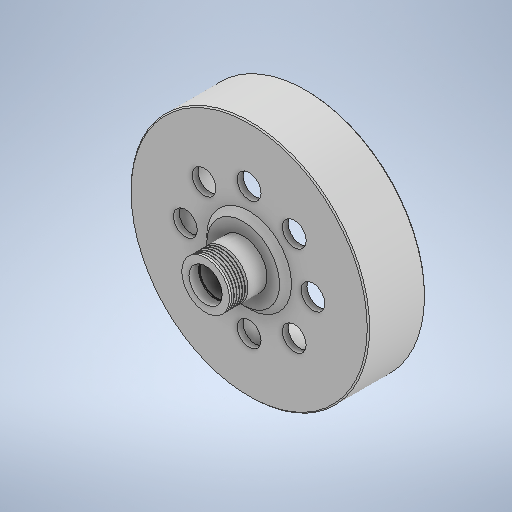
# Autodesk Inventor part: 59-01-002-B
Saved by Autodesk Inventor 2025.2 (Build 292293000, 293)
## iProperties
Created: 2024-11-28
Part Number: 59-01-002-B
Material: Generic
Document SubType Name: Modeling
Designer: Zvonko.Gabric
Density: 1 g/cm^3
Appearance: Default
Author: Zvonko.Gabric
Autodesk Inventor part; units mm, degrees
ref_plane "YZ Plane" through (0, 0, 0) normal (1, 0, 0) x (0, 1, 0)
ref_plane "XZ Plane" through (0, 0, 0) normal (0, 1, 0) x (-1, 0, 0)
ref_plane "XY Plane" through (0, 0, 0) normal (0, 0, 1) x (1, 0, 0)
sketch "Sketch1" plane through (0, 0, 0) normal (0, 1, 0) x (-1, 0, 0)
  line L0 (0, 0) -> (0, 81.9907)
  line L1 (100, 48) -> (100, 0)
  line L2 (35.5, 48) -> (100, 48)
  line L3 (30.5, 53) -> (35.5, 48)
  line L4 (20, 53) -> (30.5, 53)
  line L5 (20, 68.9767) -> (20, 53)
  line L6 (18.0006, 69.7045) -> (20, 68.9767)
  line L7 (19.8684, 70.9857) -> (18.0006, 70.3059)
  line L8 (18.0006, 72.0414) -> (19.8684, 71.3616)
  line L9 (19.8684, 73.3227) -> (18.0006, 72.6428)
  line L10 (18.0006, 74.3784) -> (19.8684, 73.6986)
  line L11 (19.8684, 75.6597) -> (18.0006, 74.9798)
  line L12 (18.0006, 76.7154) -> (19.8684, 76.0355)
  line L13 (19.8684, 77.9966) -> (18.0006, 77.3168)
  line L14 (18.0006, 79.0523) -> (19.8684, 78.3725)
  line L15 (19.8684, 80.3336) -> (18.0006, 79.6537)
  line L16 (18.0006, 81.3893) -> (19.8684, 80.7095)
  line L17 (0, 81.9907) -> (18.0006, 81.9907)
  line L18 (0, 0) -> (0, 81.9907)
  line L19 (100, 0) -> (0, 0)
  arc A0 (18.0006, 70.3059) -> (18.0006, 69.7045) centre (18.11, 70.0052) ccw
  arc A1 (19.8684, 70.9857) -> (19.8684, 71.3616) centre (19.8, 71.1737) ccw
  arc A2 (18.0006, 72.6428) -> (18.0006, 72.0414) centre (18.11, 72.3421) ccw
  arc A3 (19.8684, 73.3227) -> (19.8684, 73.6986) centre (19.8, 73.5106) ccw
  arc A4 (18.0006, 74.9798) -> (18.0006, 74.3784) centre (18.11, 74.6791) ccw
  arc A5 (19.8684, 75.6597) -> (19.8684, 76.0355) centre (19.8, 75.8476) ccw
  arc A6 (18.0006, 77.3168) -> (18.0006, 76.7154) centre (18.11, 77.0161) ccw
  arc A7 (19.8684, 77.9966) -> (19.8684, 78.3725) centre (19.8, 78.1846) ccw
  arc A8 (18.0006, 79.6537) -> (18.0006, 79.0523) centre (18.11, 79.353) ccw
  arc A9 (19.8684, 80.3336) -> (19.8684, 80.7095) centre (19.8, 80.5215) ccw
  arc A10 (18.0006, 81.9907) -> (18.0006, 81.3893) centre (18.11, 81.69) ccw
  dimension "d0" = 0
  dimension "d1" = 48
  dimension "d2" = 64.5
  dimension "d3" = 135
  dimension "d4" = 135
  dimension "d5" = 90
  dimension "d6" = 10.5
  dimension "d7" = 15.9767
  dimension "d8" = 40
  dimension "d9" = 40
  dimension "d10" = 40
  dimension "d11" = 40
  dimension "d12" = 40
  dimension "d13" = 81.9907
  dimension "d14" = 18.0006
  dimension "d15" = 0.32
  dimension "d16" = 0.32
  dimension "d17" = 0.32
  dimension "d18" = 0.32
  dimension "d19" = 0.32
  dimension "d20" = 0.32
  dimension "d21" = 100
  dimension "d22" = 0.2
  dimension "d23" = 0.2
  dimension "d24" = 0.2
  dimension "d25" = 0.2
  dimension "d26" = 0.2
  dimension "d27" = 0.3007
  dimension "d28" = 1.4692
  dimension "d29" = 2.6377
  dimension "d30" = 3.8062
  dimension "d31" = 4.9746
  dimension "d32" = 6.1431
  dimension "d33" = 7.3116
  dimension "d34" = 8.4801
  dimension "d35" = 9.6486
  dimension "d36" = 10.817
  dimension "d37" = 11.9855
  dimension "d38" = 110
  dimension "d39" = 13.014
  dimension "d40" = 1.9877
  dimension "d41" = 1.9877
  dimension "d42" = 1.9877
  dimension "d43" = 1.9877
  dimension "d44" = 1.9877
  dimension "d45" = 1.9877
  dimension "d46" = 1.9877
  dimension "d48" = 1.9877
  dimension "d49" = 1.9877
  dimension "d50" = 1.9877
  dimension "d51" = 2.1278
  dimension "d52" = 0.6014
  dimension "d53" = 1.7356
  dimension "d54" = 0.6014
  dimension "d55" = 0.6014
  dimension "d56" = 0.6014
  dimension "d57" = 0.6014
  dimension "d58" = 0.6014
  dimension "d59" = 80
  dimension "d60" = 1.89
  constraints: 40 end point, 22 point on circle, 11 centre point
  measures "d0" distance of point (0, 0) L0.start
  measures "d1" distance of L1.start L1.end
  measures "d2" distance of L2.start L1.start
  measures "d3" angle of L2 L3
  measures "d4" angle of L3 L4
  measures "d5" angle of L5 L4
  measures "d6" distance of L4.start L3.start
  measures "d7" distance of L5.start L4.start
  measures "d8" angle of L6 L7
  measures "d9" angle of L9 L8
  measures "d10" angle of L11 L10
  measures "d11" angle of L13 L12
  measures "d12" angle of L15 L14
  measures "d13" distance of L0.start L0.end
  measures "d14" distance of L0.end L17.end
  measures "d15" radius of A10
  measures "d16" radius of A8
  measures "d17" radius of A6
  measures "d18" radius of A4
  measures "d19" radius of A2
  measures "d20" radius of A0
  measures "d21" distance of L1.end L0.start
  measures "d22" radius of A9
  measures "d23" radius of A7
  measures "d24" radius of A5
  measures "d25" radius of A3
  measures "d26" radius of A1
  measures "d27" distance from line of L17 A10.centre
  measures "d28" distance from line of L17 A9.centre
  measures "d29" distance from line of L17 A8.centre
  measures "d30" distance from line of L17 A7.centre
  measures "d31" distance from line of L17 A6.centre
  measures "d32" distance from line of L17 A5.centre
  measures "d33" distance from line of L17 A4.centre
  measures "d34" distance from line of L17 A3.centre
  measures "d35" distance from line of L17 A2.centre
  measures "d36" distance from line of L17 A1.centre
  measures "d37" distance from line of L17 A0.centre
  measures "d38" angle of L5 L6
  measures "d39" distance from line of L17 L5.start
  measures "d40" distance of L16.start L16.end
  measures "d41" distance of L15.start L15.end
  measures "d42" distance of L14.start L14.end
  measures "d43" distance of L13.start L13.end
  measures "d44" distance of L12.start L12.end
  measures "d45" distance of L11.start L11.end
  measures "d46" distance of L10.start L10.end
  measures "d48" distance of L9.start L9.end
  measures "d49" distance of L8.start L8.end
  measures "d50" distance of L7.start L7.end
  measures "d51" distance of L6.start L5.start
  measures "d52" distance of L17.end L16.start
  measures "d53" distance of L15.end L16.start
  measures "d54" distance of L14.start L15.end
  measures "d55" distance of L12.start L13.end
  measures "d56" distance of L10.start L11.end
  measures "d57" distance of L8.start L9.end
  measures "d58" distance of L6.start L7.end
  measures "d59" distance between parallel lines of L1 L5
  measures "d60" distance from line of L5 A0.centre
revolve "Revolution1" add sketch "Sketch1" angle 360 about axis through (0, 0, 0) along (0, 0, 1)
sketch "Sketch2" plane through (0, 0, 0) normal (0, 0, -1) x (-1, 0, 0)
  circle A0 centre (0, 0) radius 71.8
  dimension "d62" = 143.6
  constraints: 1 centre point, 1 coincident
  measures "d62" diameter of A0
extrude "Extrusion1" cut sketch "Sketch2" against normal blind 40
sketch "Sketch3" plane through (0, 0, 0) normal (0, 0, -1) x (-1, 0, 0)
  circle A0 centre (0, 0) radius 68.8
  dimension "d65" = 137.6
  constraints: 1 centre point, 1 coincident
  measures "d65" diameter of A0
extrude "Extrusion2" cut sketch "Sketch3" against normal blind 43
sketch "Sketch4" plane through (0, 0, 0) normal (1, 0, 0) x (0, 1, 0)
  line L0 (68.8, 43) -> (-68.8, 43) projected
  line L1 (0, 43) -> (14, 43)
  line L2 (14, 43) -> (14, 37)
  line L3 (14, 37) -> (24, 37)
  line L4 (24, 37) -> (38.8, 37) construction
  line L5 (38.8, 37) -> (38.8, 43) construction
  line L6 (38.8, 43) -> (24, 37)
  line L7 (0, 43) -> (0, 33.9753) construction
  point P0 (0, 0)
  dimension "d68" = 14
  dimension "d69" = 6
  dimension "d70" = 10
  dimension "d73" = 38.8
  constraints: 14 end point, 3 perpendicular, 3 point on line, 1 midpoint, 1 vertical
  measures "d68" distance of L1.start L1.end
  measures "d69" distance of L1.end L2.end
  measures "d70" distance of L2.end L3.end
  measures "d73" distance from line of L7 L5.end
revolve "Revolution2" add sketch "Sketch4" angle 360 about axis through (0, 0, 43) along (0, 0, -1)
sketch "Sketch6" plane through (0, 0, 0) normal (0, 1, 0) x (-1, 0, 0)
  point P0 (0, 0)
sketch "Sketch7" plane through (0, 0, 0) normal (0, 1, 0) x (-1, 0, 0)
  line L0 (18.0006, 81.9907) -> (-18.0006, 81.9907) projected
  line L1 (0, 81.9907) -> (0, 82.7207)
  arc A0 (19.8684, 80.3336) -> (19.8684, 80.7095) centre (19.8, 80.5215) ccw projected
  line L2 (0, 82.7207) -> (20, 82.7207)
  line L3 (18.0006, 81.9907) -> (20, 82.7207)
  point P0 (0, 0)
  dimension "d77" = 0.73
  constraints: 6 end point, 1 midpoint, 1 vertical
  measures "d77" distance of L1.start L1.end
revolve "Revolution3" add sketch "Sketch7" angle 360 about axis through (0, 0, 81.9907) along (0, 0, 1)
sketch "Sketch8" plane through (0, 0, 82.7207) normal (0, 0, 1) x (1, 0, 0)
  circle A0 centre (0, 0) radius 20
  constraints: 1 centre point, 1 coincident
extrude "Extrusion4" add sketch "Sketch8" along normal blind 1.78
sketch "Sketch9" plane through (0, 0, 0) normal (0, 1, 0) x (-1, 0, 0)
  line L0 (20, 84.5007) -> (-20, 84.5007) projected
  line L1 (0, 84.5007) -> (0, 37.0007)
  line L2 (0, 37.0007) -> (10.9209, 37.0007)
  line L3 (0, 37.0007) -> (14, 37)
  line L4 (-14, 37) -> (14, 37) projected
  line L5 (14, 37) -> (14, 75.2)
  line L6 (13.9351, 75.2) -> (14.6351, 75.2)
  line L7 (19.8684, 75.6597) -> (-19.8684, 75.6597) projected
  line L8 (14.6351, 75.2) -> (14.6351, 76.5)
  line L9 (14.6351, 76.5) -> (13.9351, 76.5)
  line L10 (13.9351, 76.5) -> (13.9351, 84.5007)
  line L11 (0, 84.5007) -> (13.9351, 84.5007)
  point P0 (0, 0)
  dimension "d81" = 47.5
  dimension "d82" = 14
  dimension "d83" = 38.2
  dimension "d84" = 0.7
  dimension "d86" = 1.3
  dimension "d87" = 0.7
  constraints: 19 end point, 3 vertical, 2 horizontal, 2 perpendicular, 1 collinear, 1 midpoint, 1 point on line
  measures "d81" distance of L1.start L1.end
  measures "d82" distance of L1.end L3.end
  measures "d83" distance of L3.end L5.end
  measures "d84" distance of L6.start L6.end
  measures "d86" distance of L6.end L8.end
  measures "d87" distance of L8.end L9.end
revolve "Revolution4" cut sketch "Sketch9" angle 360 about axis through (0, 0, 84.5007) along (0, 0, -1)
sketch "Sketch10" plane through (0, 0, 48) normal (0, 0, 1) x (1, 0, 0)
  circle A0 centre (0, 0) radius 13.9351 projected
  circle A1 centre (0, 0) radius 53.5 construction
  circle A2 centre (-53.5, 0) radius 10
  circle A3 centre (0, 0) radius 53.5 construction
  circle A4 centre (-37.8302, -37.8302) radius 10
  circle A5 centre (0, 0) radius 53.5 construction
  circle A6 centre (0, -53.5) radius 10
  circle A7 centre (0, 0) radius 53.5 construction
  circle A8 centre (37.8302, -37.8302) radius 10
  circle A9 centre (0, 0) radius 53.5 construction
  circle A10 centre (53.5, 0) radius 10
  circle A11 centre (0, 0) radius 53.5 construction
  circle A12 centre (37.8302, 37.8302) radius 10
  circle A13 centre (0, 0) radius 53.5 construction
  circle A14 centre (0, 53.5) radius 10
  circle A15 centre (0, 0) radius 53.5 construction
  circle A16 centre (-37.8302, 37.8302) radius 10
  line L0 (-53.5, 0) -> (-35.5, 0) construction
  circle A17 centre (0, 0) radius 35.5 projected
  circle A18 centre (0, 0) radius 38.8 projected
  line L1 (-37.8302, -37.8302) -> (0, 0) construction
  dimension "d89" = 107
  dimension "d90" = 20
  dimension "d93" = 360
  constraints: 9 centre point, 4 end point, 3 coincident, 3 horizontal alignment, 2 coincident with centre, 2 point on circle, 2 vertical alignment, 1 horizontal, 47 other
  measures "d90" diameter of A2
extrude "Extrusion5" cut sketch "Sketch10" against normal blind 10 contours A2 | A4 | A6 | A8 | A10 | A12 | A14 | A16
chamfer "Chamfer1" distance 1 angle 45 1 edges at (100, 0, 0) measured on face at (-57.1537, 70.0144, 0)
chamfer "Chamfer2" distance 1 angle 45 1 edges at (100, 0, 48) measured on face at (-66.0249, 28.1135, 48)
body "Solid1"
